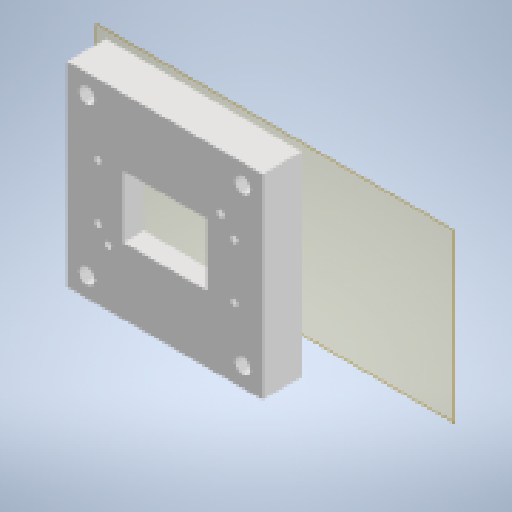
# Autodesk Inventor part: mocowanie_2000
Saved by Autodesk Inventor 2025.1 (Build 291241000, 241)
## iProperties
Created: 2024-10-24
Part Number: mocowanie_2000
Material: Ogólny
Document SubType Name: Modeling
Designer: PC
Density: 1 g/cm^3
Appearance: Domyślna
Author: PC
Autodesk Inventor part; units mm, degrees
ref_plane "YZ Plane" through (0, 0, 0) normal (1, 0, 0) x (0, 1, 0)
ref_plane "XZ Plane" through (0, 0, 0) normal (0, 1, 0) x (-1, 0, 0)
ref_plane "XY Plane" through (0, 0, 0) normal (0, 0, 1) x (1, 0, 0)
ref_plane "Płaszczyzna konstrukcyjna1" through (0, 0, 0) normal (0, 0, 1) x (1, 0, 0)
sketch "Szkic1" plane through (0, 0, 0) normal (0, 0, 1) x (1, 0, 0)
  circle A0 centre (-0.75, -19.05) radius 2 projected
  circle A1 centre (-0.75, 1.9) radius 2 projected
  circle A2 centre (-53.2, 1.9) radius 2 projected
  circle A3 centre (-53.2, -19.05) radius 2 projected
  arc A4 (-7.07, 6.8616) -> (-7.3, 7.3) centre (-6.1, 7.65) ccw projected
  line L0 (-7.07, 6.8616) -> (-7.07, -24.52) projected
  line L1 (-7.07, -24.52) -> (-47.8, -24.52) projected
  line L2 (-47.8, -24.52) -> (-47.8, 7.3) projected
  line L3 (-47.8, 7.3) -> (-7.3, 7.3) projected
  arc A5 (-49.8576, -25.4424) -> (-50.3424, -24.9576) centre (-49.25, -24.35) ccw projected
  line L4 (-49.8576, -25.4424) -> (-47.9, -27.4) projected
  line L5 (-47.9, -27.4) -> (-33.9, -27.4) projected
  line L6 (-33.9, -27.4) -> (-30.0895, -29.6) projected
  line L7 (-30.0895, -29.6) -> (-13.35, -29.6) projected
  line L8 (-13.35, -29.6) -> (-11.15, -27.4) projected
  line L9 (-11.15, -27.4) -> (-7.15, -27.4) projected
  line L10 (-7.15, -27.4) -> (-2.65, -22.9) projected
  line L11 (-2.65, -22.9) -> (-2.65, 6.4) projected
  line L12 (-2.65, 6.4) -> (-6.65, 10.4) projected
  line L13 (-6.65, 10.4) -> (-47.9, 10.4) projected
  arc A6 (-47.9, 10.4) -> (-50.9, 7.4) centre (-47.9, 7.4) ccw projected
  line L14 (-50.9, 7.4) -> (-50.9, -24.4) projected
  line L15 (-50.9, -24.4) -> (-50.3424, -24.9576) projected
  line L16 (-50.3424, -24.9576) -> (-49.8576, -25.4424) projected
  arc A7 (-49.8576, -25.4424) -> (-50.3424, -24.9576) centre (-49.25, -24.35) ccw projected
  line L17 (-42.875, -20.03) -> (-42.875, 2.83) projected
  line L18 (-42.875, 2.83) -> (-12.075, 2.83) projected
  line L19 (-12.075, 2.83) -> (-12.075, -20.03) projected
  line L20 (-12.075, -20.03) -> (-42.875, -20.03) projected
  line L21 (-45.382, -22.57) -> (-9.568, -22.57) projected
  line L22 (-9.568, -22.57) -> (-9.568, 5.37) projected
  line L23 (-9.568, 5.37) -> (-45.382, 5.37) projected
  line L24 (-45.382, 5.37) -> (-45.382, -22.57) projected
  arc A8 (-18.975, -17.3) -> (-14.775, -13.1) centre (-18.975, -13.1) ccw projected
  line L25 (-18.975, -17.3) -> (-35.975, -17.3) projected
  arc A9 (-40.175, -13.1) -> (-35.975, -17.3) centre (-35.975, -13.1) ccw projected
  line L26 (-40.175, -13.1) -> (-40.175, -4.1) projected
  arc A10 (-35.975, 0.1) -> (-40.175, -4.1) centre (-35.975, -4.1) ccw projected
  line L27 (-35.975, 0.1) -> (-18.975, 0.1) projected
  arc A11 (-14.775, -4.1) -> (-18.975, 0.1) centre (-18.975, -4.1) ccw projected
  line L28 (-14.775, -4.1) -> (-14.775, -13.1) projected
  line L29 (-42.875, -20.03) -> (-12.075, -20.03) projected
  line L30 (-12.075, -20.03) -> (-12.075, 2.83) projected
  line L31 (-12.075, 2.83) -> (-42.875, 2.83) projected
  line L32 (-42.875, 2.83) -> (-42.875, -20.03) projected
  line L33 (-62.5, -30.65) -> (-6.9, -30.65) construction
  line L34 (-62.5, 29.05) -> (-62.5, -29.05) projected
  line L35 (-62.5, -29.05) -> (8.2, -29.05) projected
  circle A12 centre (-0.75, -19.05) radius 1.25
  circle A13 centre (-0.75, 1.9) radius 1.25
  circle A14 centre (-53.2, 1.9) radius 1.25
  circle A15 centre (-53.2, -19.05) radius 1.25
  circle A16 centre (-49.25, -24.35) radius 1.3
  circle A17 centre (-6.1, 7.65) radius 1.3
  line L36 (-11.575, -20.53) -> (-43.375, -20.53)
  line L37 (-43.375, -20.53) -> (-43.375, 3.33)
  line L38 (-43.375, 3.33) -> (-11.575, 3.33)
  line L39 (-11.575, 3.33) -> (-11.575, -20.53)
  line L40 (-27.475, -20.03) -> (-27.475, 2.83) construction
  line L41 (-11.575, -8.6) -> (-43.375, -8.6) construction
  line L42 (2.525, -38.6) -> (-57.475, -38.6) construction
  line L43 (-57.475, -38.6) -> (-57.475, 21.4) construction
  line L44 (-57.475, 21.4) -> (2.525, 21.4) construction
  line L45 (2.525, 21.4) -> (2.525, -38.6) construction
  line L46 (2.525, -38.6) -> (-57.475, 21.4) construction
  line L47 (-57.475, -38.6) -> (2.525, 21.4) construction
  line L48 (10.025, -46.1) -> (-64.975, -46.1)
  line L49 (-64.975, -46.1) -> (-64.975, 28.9)
  line L50 (-64.975, 28.9) -> (10.025, 28.9)
  line L51 (10.025, 28.9) -> (10.025, -46.1)
  line L52 (10.025, -46.1) -> (-64.975, 28.9) construction
  line L53 (-64.975, -46.1) -> (10.025, 28.9) construction
  circle A18 centre (-57.475, 21.4) radius 3
  circle A19 centre (2.525, 21.4) radius 3
  circle A20 centre (2.525, -38.6) radius 3
  circle A21 centre (-57.475, -38.6) radius 3
  line L54 (-2.35, -32.15) -> (-51.2, -32.15)
  line L55 (-51.2, -32.15) -> (-51.2, 10.7)
  line L56 (-51.2, 10.7) -> (-2.35, 10.7)
  line L57 (-2.35, 10.7) -> (-2.35, -32.15)
  line L58 (-62.5, -32.15) -> (147.5, -32.15) projected
  point P0 (0, 0)
  point P1 (-27.475, -8.6)
  dimension "d0" = 2.5
  dimension "d1" = 2.6
  dimension "d2" = 2.6
  dimension "d3" = 0.5
  dimension "d4" = 0.5
  dimension "d5" = 0.5
  dimension "d6" = 0.5
  dimension "d7" = 60
  dimension "d8" = 75
  dimension "d9" = 6
  dimension "d10" = 0.3
  dimension "d11" = 0.3
  dimension "d12" = 0.3
  constraints: 44 end point, 10 centre point, 10 coincident, 9 midpoint, 8 parallel, 6 equal radius, 6 perpendicular, 4 horizontal, 1 collinear
  measures "d0" diameter of A12
  measures "d1" diameter of A16
  measures "d2" diameter of A17
  measures "d3" distance between parallel lines of L20 L36
  measures "d4" distance between parallel lines of L38 L31
  measures "d5" distance between parallel lines of L17 L37
  measures "d6" distance between parallel lines of L19 L39
  measures "d7" distance of L43.end L44.end
  measures "d8" distance of L49.end L50.end
  measures "d9" diameter of A18
  measures "d10" distance between parallel lines of L13 L56
  measures "d11" distance between parallel lines of L11 L57
  measures "d12" distance between parallel lines of L14 L55
extrude "Wyciągnięcie proste1" add sketch "Szkic1" along normal blind 15 contours A0 L57 | A3 | A2 | A0 L57 A1 L56 L55 L35 L34 L50 L51 L58 | L57 A0 L11 | A0 L11 A1 L57 | L57 L35 L8 L9 L10 L11 A0 | L11 A0 | A0 L11 L10 L9 L8 L35 L6 L5 L4 A16 L15 L14 A6 L13 L12 A1 | L57 A1 | A1 L11 L57 | L57 L54 L55 L35 L6 L7 L8 | A1 L11 | A1 L11 L12 L13 A6 L14 L15 A16 L4 L5 L6 L35 L55 L56 L57 | L8 L7 L6 L35 | L58 L51 L48 L49 L50 L34 L35 L55 L54 | L0 L1 L2 L3 A17 | L24 L23 L22 L21
sketch "Szkic2" plane through (0, 0, 0) normal (0, 0, -1) x (-1, 0, 0)
  line L0 (64.975, 28.9) -> (64.975, -46.1) projected
  line L1 (-10.025, 28.9) -> (64.975, 28.9) projected
  line L2 (-10.025, -46.1) -> (-10.025, 28.9) projected
  line L3 (64.975, -46.1) -> (-10.025, -46.1) projected
  line L4 (11.575, -20.53) -> (43.375, -20.53) projected
  line L5 (11.575, 3.33) -> (11.575, -20.53) projected
  line L6 (43.375, 3.33) -> (11.575, 3.33) projected
  line L7 (43.375, -20.53) -> (43.375, 3.33) projected
  circle A0 centre (49.25, -24.35) radius 1.3 projected
  circle A1 centre (57.475, -38.6) radius 3 projected
  circle A2 centre (-2.525, -38.6) radius 3 projected
  circle A3 centre (-2.525, 21.4) radius 3 projected
  circle A4 centre (57.475, 21.4) radius 3 projected
  circle A5 centre (0.75, 1.9) radius 1.25 projected
  circle A6 centre (0.75, -19.05) radius 1.25 projected
  circle A7 centre (53.2, -19.05) radius 1.25 projected
  circle A8 centre (53.2, 1.9) radius 1.25 projected
  circle A9 centre (6.1, 7.65) radius 1.3 projected
  line L8 (6.65, 10.4) -> (47.9, 10.4) projected
  arc A10 (50.9, 7.4) -> (47.9, 10.4) centre (47.9, 7.4) ccw projected
  line L9 (50.9, 7.4) -> (50.9, -24.4) projected
  line L10 (2.65, 6.4) -> (6.65, 10.4) projected
  line L11 (2.65, -22.9) -> (2.65, 6.4) projected
  line L12 (7.15, -27.4) -> (2.65, -22.9) projected
  line L13 (11.15, -27.4) -> (7.15, -27.4) projected
  line L14 (13.35, -29.6) -> (11.15, -27.4) projected
  line L15 (50.9, -24.4) -> (47.9, -27.4) projected
  line L16 (47.9, -27.4) -> (33.9, -27.4) projected
  line L17 (33.9, -27.4) -> (30.0895, -29.6) projected
  line L18 (30.0895, -29.6) -> (13.35, -29.6) projected
  line L19 (2.35, 10.7) -> (51.2, 10.7)
  line L20 (51.2, 10.7) -> (51.2, -34.4144)
  line L21 (51.2, -34.4144) -> (2.35, -34.4144)
  line L22 (2.35, -34.4144) -> (2.35, 10.7)
  line L23 (62.5, -30.65) -> (6.9, -30.65) construction
  line L24 (62.5, -32.15) -> (-147.5, -32.15) construction
  point P0 (0, 0)
  dimension "d15" = 0.3
  dimension "d16" = 0.3
  dimension "d17" = 0.3
  constraints: 8 end point, 2 parallel, 1 horizontal, 1 perpendicular
  measures "d15" distance between parallel lines of L9 L20
  measures "d16" distance between parallel lines of L8 L19
  measures "d17" distance between parallel lines of L22 L11
extrude "Wyciągnięcie proste2" cut sketch "Szkic2" against normal blind 4.33 contours A0 L15 L16 L17 L18 L14 L13 L12 L11 L10 L8 A10 L9 | L19 L20 L21 L22
